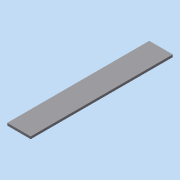
# Autodesk Inventor part: bottomplate
Saved by Autodesk Inventor 2016 (Build 200138000, 138)
## iProperties
Created: 2017-03-05
Part Number: bottomplate
Material: Generic
Document SubType Name: Modeling
Designer: Errrm
Density: 1 g/cm^3
Appearance: Default
Author: Errrm
Autodesk Inventor part; units mm, degrees
ref_plane "YZ Plane" through (0, 0, 0) normal (1, 0, 0) x (0, 1, 0)
ref_plane "XZ Plane" through (0, 0, 0) normal (0, 1, 0) x (-1, 0, 0)
ref_plane "XY Plane" through (0, 0, 0) normal (0, 0, 1) x (1, 0, 0)
sketch "Sketch1" plane through (0, 0, 0) normal (0, 0, 1) x (1, 0, 0)
  line L0 (0, 6) -> (50, 6) projected
  line L1 (50, -296) -> (0, -296) projected
  line L2 (50, -296) -> (50, 6)
  line L3 (0, 6) -> (0, -296)
  constraints: 4 end point, 1 parallel, 1 vertical
extrude "Extrusion1" add sketch "Sketch1" along normal blind 5
body "Solid1"
